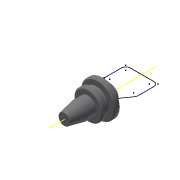
# Autodesk Inventor part: dipstick
Saved by Autodesk Inventor 2022 Beta2 (Build 260130000, 130) ContinuousBuild 0
## iProperties
Created: 2007-02-12
Part Number: dipstick
Document SubType Name: Modeling
Designer: jmacmillan
Density: 1 g/cm^3
Material: Generic
Appearance: Light Gray
Author: jmacmillan
Autodesk Inventor part; units mm, degrees
ref_plane "YZ Plane" through (0, 0, 0) normal (1, 0, 0) x (0, 1, 0)
ref_plane "XZ Plane" through (0, 0, 0) normal (0, 1, 0) x (-1, 0, 0)
sketch "Sketch1" plane through (0, 0, 0) normal (0, 0, 1) x (1, 0, 0)
  line L0 (4.0981, 21.1554) -> (4.0981, 18.0855)
  line L1 (4.0981, 18.0855) -> (7.5818, 18.0855)
  line L2 (8.0818, 17.5855) -> (8.0818, 15.9599)
  line L3 (7.5818, 15.4599) -> (0, 15.4599)
  arc A0 (4.9585, 13.4599) -> (4.9585, 15.4599) centre (4.9585, 14.4599) ccw
  line L4 (4.9585, 13.4599) -> (6.1918, 13.4599)
  line L5 (6.6918, 12.9599) -> (6.6918, 11.4899)
  line L6 (6.1918, 10.9899) -> (4.0981, 10.9899)
  line L7 (4.0981, 10.9899) -> (4.0981, 6.9999)
  line L8 (4.0981, 6.9999) -> (2.6219, 0)
  line L9 (2.6219, 0) -> (0, 0)
  line L10 (0, 21.1554) -> (4.0981, 21.1554)
  line L11 (0, 21.1554) -> (0, 0)
  line L12 (0, 28.6278) -> (0, -8.3179) projected
  line L13 (-1.6164, 0) -> (9.6982, 0) projected
  line L14 (0, 23.3498) -> (0, -3.0399)
  line L15 (8.0818, 17.5855) -> (7.5818, 18.0855)
  line L16 (6.6918, 12.9599) -> (6.1918, 13.4599)
  line L17 (6.1918, 10.9899) -> (6.6918, 11.4899)
  line L18 (7.5818, 15.4599) -> (8.0818, 15.9599)
  point P0 (8.0818, 18.0855)
  point P1 (8.0818, 15.4599)
  point P2 (6.6918, 13.4599)
  point P3 (6.6918, 10.9899)
  point P4 (8.0818, 18.0855)
  point P5 (8.0818, 15.4599)
  point P6 (6.6918, 13.4599)
  point P7 (6.6918, 10.9899)
  point P8 (8.0818, 15.4599)
  dimension "d22" = 0.5
  dimension "d23" = 45
  dimension "d31" = 4.0981
  dimension "d32" = 8.0818
  dimension "d33" = 6.6918
  dimension "d34" = 2.6219
  dimension "d36" = 6.9999
  dimension "d37" = 10.9899
  dimension "d38" = 2.47
  dimension "d39" = 2.6256
  dimension "d40" = 1
  constraints: 34 end point, 22 point on line, 6 parallel, 4 collinear, 3 equal length, 2 perpendicular, 2 point on circle, 2 tangent, 1 centre point
  measures "d22" distance of L2.start point (8.082, 18.085)
  measures "d23" angle of L2 L15
  measures "d31" distance between parallel lines of L11 L0
  measures "d32" distance between parallel lines of L14 L2
  measures "d33" distance between parallel lines of L12 L5
  measures "d34" distance from line of L11 L8.end
  measures "d36" distance from line of L7.end L9
  measures "d37" distance between parallel lines of L6 L9
  measures "d38" distance between parallel lines of L4 L6
  measures "d39" distance between parallel lines of L1 L3
  measures "d40" radius of A0
revolve "Revolution1" add sketch "Sketch1" angle 360 about axis through (0, 23.3498, 0) along (0, -1, 0)
sketch "Handle Path" plane through (0, 0, 0) normal (0, 0, 1) x (1, 0, 0)
  line L0 (-2.5861, 18.9963) -> (-7.1383, 25.4974)
  line L1 (-7.5, 26.6446) -> (-7.5, 34.014)
  line L2 (-5.5, 36.014) -> (5.5, 36.014)
  line L3 (7.5, 34.014) -> (7.5, 26.6446)
  line L4 (7.1383, 25.4974) -> (2.5861, 18.9963)
  line L5 (0, 42.6716) -> (0, -7.1119) projected
  arc A0 (-7.5, 26.6446) -> (-7.1383, 25.4974) centre (-5.5, 26.6446) ccw
  arc A1 (-5.5, 36.014) -> (-7.5, 34.014) centre (-5.5, 34.014) ccw
  arc A2 (7.5, 34.014) -> (5.5, 36.014) centre (5.5, 34.014) ccw
  arc A3 (7.1383, 25.4974) -> (7.5, 26.6446) centre (5.5, 26.6446) ccw
  point P0 (-7.5, 26.014)
  point P1 (-7.5, 36.014)
  point P2 (7.5, 36.014)
  dimension "d43" = 15
  dimension "d44" = 10
  dimension "d47" = 35
  dimension "d49" = 2
  dimension "d51" = 5.1723
  constraints: 10 end point, 8 point on circle, 8 tangent, 6 point on line, 4 centre point, 3 equal radius, 2 perpendicular, 1 symmetric about line, 2 other
  measures "d43" distance of point (-7.5, 36.014) point (7.5, 36.014)
  measures "d44" distance of point (-7.5, 26.014) point (-7.5, 36.014)
  measures "d47" angle of L5 L0
  measures "d49" radius of A0
  measures "d51" distance of L4.end L0.start
ref_plane "Work Plane2" through (-2.5861, 18.9963, 0) normal (-0.5736, 0.8192, 0) x (-0.8192, -0.5736, 0)
sketch "Handle Profile" plane through (-2.5861, 18.9963, 0) normal (-0.5736, 0.8192, 0) x (-0.8192, -0.5736, 0)
  circle A0 centre (0, 0) radius 0.9741
  dimension "d48" = 1.9483
  constraints: 1 centre point
  measures "d48" diameter of A0
body "Solid1"
